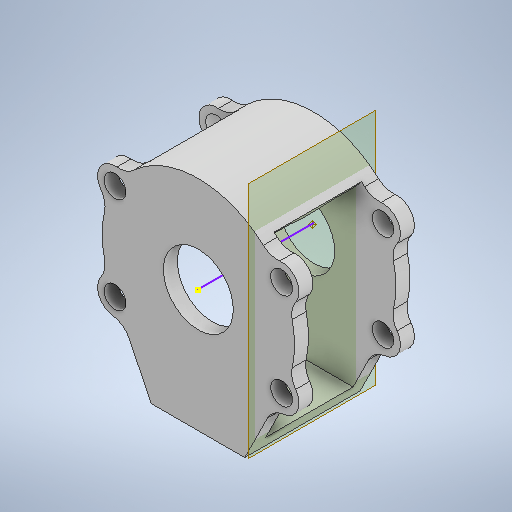
# Autodesk Inventor part: pulleyblocker
Saved by Autodesk Inventor 2025.2 (Build 292293000, 293)
## iProperties
Created: 2025-01-13
Part Number: pulleyblocker
Material: Generic
Document SubType Name: Modeling
Designer: email
Density: 1 g/cm^3
Appearance: Default
Author: email
Autodesk Inventor part; units mm, degrees
ref_plane "YZ Plane" through (0, 0, 0) normal (1, 0, 0) x (0, 1, 0)
ref_plane "XZ Plane" through (0, 0, 0) normal (0, 1, 0) x (-1, 0, 0)
ref_plane "XY Plane" through (0, 0, 0) normal (0, 0, 1) x (1, 0, 0)
sketch "Sketch1" plane through (0, 0, 0) normal (0, 0, 1) x (1, 0, 0)
  line L0 (-13.5571, -30) -> (11.7429, -30) construction
  line L1 (11.7429, -30) -> (11.7429, -13.7014) construction
  line L2 (11.7429, -13.7014) -> (-13.5571, -13.7014) construction
  line L3 (-13.5571, -13.7014) -> (-13.5571, -30) construction
  circle A0 centre (0, 0) radius 10
  circle A1 centre (0, 0) radius 23.5 construction
  line L4 (11.7429, -30) -> (21.2173, -10.1032) construction
  line L5 (-13.5571, -30) -> (-21.9053, -8.5093) construction
  circle A2 centre (0, 0) radius 27.5
  line L6 (-13.4496, -35) -> (13.2752, -35)
  line L7 (-13.4496, -35) -> (-24.6844, -12.1216)
  line L8 (13.2752, -35) -> (24.6094, -12.273)
  circle A3 centre (23.8157, 13.75) radius 5
  line L9 (-0.006, -0.0035) -> (23.8157, 13.75) construction
  line L10 (-0.006, -0.0035) -> (30.724, -0.0035) construction
  line L11 (-0.006, -0.0035) -> (23.8127, -13.7552) construction
  circle A4 centre (23.8127, -13.7552) radius 5
  circle A5 centre (23.8157, 13.75) radius 3.075
  circle A6 centre (23.8127, -13.7552) radius 3.075
  line L12 (-0.006, -0.0035) -> (-0.006, 21.9972)
  circle A7 centre (-23.8278, 13.75) radius 5
  circle A8 centre (-23.8248, -13.7552) radius 5
  circle A9 centre (-23.8278, 13.75) radius 3.075
  circle A10 centre (-23.8248, -13.7552) radius 3.075
  point P0 (20.9324, 17.8349)
  point P1 (-20.9369, 17.8296)
  point P2 (-25.9134, 9.2058)
  point P3 (-25.9114, -9.2114)
  point P4 (-21.6672, -18.2658)
  point P5 (21.6274, -18.2524)
  point P6 (25.9097, -9.2162)
  point P7 (25.9117, 9.2105)
  dimension "d0" = 25.3
  dimension "d1" = 20
  dimension "d2" = 30
  dimension "d3" = 47
  dimension "d4" = 55
  dimension "d5" = 5
  dimension "d45" = 30
  dimension "d46" = 10
  dimension "d47" = 30
  dimension "d48" = 10
  dimension "d49" = 6.15
  dimension "d50" = 6.15
  dimension "d64" = 6.15
  constraints: 26 end point, 11 centre point, 8 coincident, 6 point on circle, 4 symmetric about line, 4 tangent, 3 horizontal, 2 parallel, 1 perpendicular, 1 point on line, 1 vertical, 4 other
  measures "d0" distance between parallel lines of L1 L3
  measures "d1" diameter of A0
  measures "d2" distance from line of L0 A0.centre
  measures "d3" diameter of A1
  measures "d4" diameter of A2
  measures "d5" distance between parallel lines of L6 L0
  measures "d45" angle of L10 L9
  measures "d46" diameter of A3
  measures "d47" angle of L10 L11
  measures "d48" diameter of A4
  measures "d49" diameter of A5
  measures "d50" diameter of A6
  measures "d64" diameter of A9
extrude "Extrusion1" add sketch "Sketch1" along normal blind 4 contours A2 A4 A8 A7 A3 | A3 A2 A5 | A2 A5 A3 | A4 L8 A6 A2 | A2 A6 A4 | A4 L8 L6 L7 A8 A2 | A2 A6 L8 A4 | A7 A2 A9 | A2 A9 A7 | A8 L7 A10 A2 | A2 A10 A8 | A8 A2 A10 L7
sketch "Sketch2" plane through (0, 0, 4) normal (0, 0, 1) x (1, 0, 0)
  line L0 (-21.6672, -18.2658) -> (-13.4496, -35) projected
  line L1 (-13.4496, -35) -> (-15.4139, -31)
  line L2 (15.2701, -31) -> (-15.4139, -31)
  line L3 (13.2752, -35) -> (21.6274, -18.2524) projected
  line L4 (15.2701, -31) -> (13.2752, -35)
  line L5 (-13.4496, -35) -> (13.2752, -35) projected
  line L6 (-13.4496, -35) -> (13.2752, -35)
  point P0 (0, 0)
  point P1 (-24.6844, -12.1216)
  point P2 (24.6094, -12.273)
  dimension "d8" = 4
  constraints: 8 end point, 2 collinear, 2 point on line, 1 horizontal
  measures "d8" distance between parallel lines of L5 L2
extrude "Extrusion2" add sketch "Sketch2" along normal blind 25
sketch "Sketch3" plane through (0, 0, 29) normal (0, 0, 1) x (1, 0, 0)
  line L0 (-13.5571, -30) -> (11.7429, -30) construction
  line L1 (11.7429, -30) -> (11.7429, -13.7014) construction
  line L2 (11.7429, -13.7014) -> (-13.5571, -13.7014) construction
  line L3 (-13.5571, -13.7014) -> (-13.5571, -30) construction
  circle A0 centre (0, 0) radius 10
  circle A1 centre (0, 0) radius 23.5 construction
  line L4 (11.7429, -30) -> (21.2173, -10.1032) construction
  line L5 (-13.5571, -30) -> (-21.9053, -8.5093) construction
  circle A2 centre (0, 0) radius 27.5
  line L6 (-13.4496, -35) -> (13.2752, -35)
  line L7 (-13.4496, -35) -> (-24.6844, -12.1216)
  line L8 (13.2752, -35) -> (24.6094, -12.273)
  circle A3 centre (23.8157, 13.75) radius 5
  line L9 (-0.006, -0.0035) -> (23.8157, 13.75) construction
  line L10 (-0.006, -0.0035) -> (30.724, -0.0035) construction
  line L11 (-0.006, -0.0035) -> (23.8127, -13.7552) construction
  circle A4 centre (23.8127, -13.7552) radius 5
  circle A5 centre (23.8157, 13.75) radius 3.125
  circle A6 centre (23.8127, -13.7552) radius 3.125
  line L12 (-0.006, -0.0035) -> (-0.006, 21.9972)
  circle A7 centre (-23.8278, 13.75) radius 5
  circle A8 centre (-23.8278, 13.75) radius 3.125
  circle A9 centre (-23.8248, -13.7552) radius 5
  circle A10 centre (-23.8248, -13.7552) radius 3.125
  circle A11 centre (0, 0) radius 10 projected
  point P0 (-42.8581, 50.0798)
  point P1 (-84.7274, 50.0745)
  point P2 (-89.7039, 41.4507)
  point P3 (-89.7018, 23.0335)
  point P4 (-85.4577, 13.9792)
  point P5 (-42.163, 13.9925)
  point P6 (-37.8808, 23.0287)
  point P7 (-37.8788, 41.4554)
  point P8 (20.9324, 17.8349)
  point P9 (-20.9369, 17.8296)
  point P10 (-25.9134, 9.2058)
  point P11 (-25.9114, -9.2114)
  point P12 (-21.6672, -18.2658)
  point P13 (21.6274, -18.2524)
  point P14 (20.9285, -17.8395)
  point P15 (22.0984, -16.368)
  point P16 (25.2195, -10.9648)
  point P17 (25.9117, 9.2105)
  point P18 (25.9097, -9.2162)
  dimension "d51" = 25.3
  dimension "d52" = 20
  dimension "d53" = 30
  dimension "d54" = 47
  dimension "d55" = 55
  dimension "d56" = 5
  dimension "d57" = 30
  dimension "d58" = 10
  dimension "d59" = 30
  dimension "d60" = 10
  dimension "d61" = 6.25
  dimension "d62" = 6.25
  constraints: 26 end point, 11 centre point, 8 coincident, 6 point on circle, 4 symmetric about line, 4 tangent, 3 horizontal, 2 parallel, 1 concentric, 1 perpendicular, 1 point on line, 1 vertical, 4 other
  measures "d51" distance between parallel lines of L1 L3
  measures "d52" diameter of A0
  measures "d53" distance from line of L0 A0.centre
  measures "d54" diameter of A1
  measures "d55" diameter of A2
  measures "d56" distance between parallel lines of L6 L0
  measures "d57" angle of L10 L9
  measures "d58" diameter of A3
  measures "d59" angle of L10 L11
  measures "d60" diameter of A4
  measures "d61" diameter of A5
  measures "d62" diameter of A6
extrude "Extrusion3" add sketch "Sketch3" along normal blind 4 contours A2 A4 A9 A7 A3 | A3 A2 A5 | A2 A5 A3 | A4 L8 A6 A2 | A2 A6 A4 | A4 L8 L6 L7 A9 A2 | A2 A6 L8 A4 | A7 A2 A8 | A2 A8 A7 | A9 L7 A10 A2 | A2 A10 A9 | A9 A2 A10 L7
sketch "Sketch4" plane through (0, 0, 0) normal (1, 0, 0) x (0, 1, 0)
  line L0 (-31, 4) -> (-31, 29) projected
  line L1 (16.3793, 67.7391) -> (20.3793, 67.7391) construction
  line L2 (20.3793, 44.4757) -> (20.3793, 67.7391) construction
  line L3 (20.3793, 44.4757) -> (16.3793, 44.4757) construction
  line L4 (0, 24) -> (0, 4)
  line L5 (16.3793, 44.4757) -> (16.3793, 48.4757) construction
  line L6 (16.3793, 67.7391) -> (16.3793, 63.7391) construction
  arc A0 (16.3793, 63.7391) -> (16.3793, 48.4757) centre (22.0199, 56.1074) ccw construction
  line L7 (27.5, 4) -> (17.8296, 4) projected
  line L8 (27.5, 29) -> (27.5, 33)
  line L9 (27.5, 29) -> (-12.273, 29)
  line L10 (27.5, 29) -> (25, 29)
  line L11 (25, 29) -> (25, 22.5)
  arc A1 (25, 22.5) -> (25, 10.5) centre (31.0208, 16.5) ccw
  line L12 (25, 10.5) -> (25, 4)
  line L13 (27.5, 4) -> (25, 4)
  line L14 (25, 29) -> (27.5, 29)
  line L15 (27.5, 4) -> (27.5, 29)
  line L16 (27.5, 4) -> (17.8296, 4) projected
  line L17 (27.5, 4) -> (25, 4)
  point P0 (0, 0)
  point P1 (-12.1216, 29)
  point P2 (-12.1216, 4)
  point P3 (-12.273, 29)
  point P4 (25, 7.25)
  point P5 (17.8349, 4)
  point P6 (9.2058, 4)
  point P7 (-9.2114, 4)
  dimension "d22" = 4
  dimension "d23" = 4
  dimension "d24" = 4
  dimension "d26" = 6.5
  dimension "d28" = 6.5
  dimension "d65" = 2.5
  dimension "d66" = 2.5
  constraints: 28 end point, 4 collinear, 4 point on circle, 3 perpendicular, 3 vertical, 2 centre point, 2 point on line, 1 coincident, 1 horizontal, 1 midpoint, 4 other
  measures "d22" distance of L3.end L5.end
  measures "d23" distance of L1.start L6.end
  measures "d24" distance between parallel lines of L2 L5
  measures "d26" distance of L10.end L11.end
  measures "d28" distance of L12.start L12.end
  measures "d65" distance between parallel lines of L15 L11
  measures "d66" distance between parallel lines of L15 L12
revolve "Revolution1" add sketch "Sketch4" angle 80 mid plane about axis through (0, 0, 24) along (0, 0, -1)
sketch "Sketch5" plane through (0, 0, 0) normal (0, 1, 0) x (-1, 0, 0)
  line L0 (0, 0) -> (0.0872, 33)
  constraints: 2 end point
sketch "Sketch7" plane through (0, 0, 0) normal (1, 0, 0) x (0, 1, 0)
  line L0 (29.2747, 11.9493) -> (29.2747, 21.0264) construction
  ellipse E0 centre (23.7633, 16.5) end of major axis (23.7633, 8) minor radius 6.5114 (19.1511, 22.5) -> (19.1511, 10.5) ccw projected
  line L1 (29.2747, 16.4878) -> (30.2747, 16.4878)
  arc A0 (29.2747, 11.9493) -> (29.2747, 21.0264) centre (45.8325, 16.4878) ccw
  arc A1 (30.2415, 15.6424) -> (30.2747, 16.4878) centre (23.4449, 16.3328) ccw
  line L2 (29.2747, 21.0264) -> (27.6139, 21.0264)
  line L3 (27.6139, 21.0264) -> (27.6139, 13.9093)
  line L4 (27.6139, 13.9093) -> (29.2747, 13.9093)
  line L5 (29.2747, 13.9093) -> (29.2747, 21.0264)
  point P0 (0, 0)
  point P1 (13.8599, 14.7128)
  point P2 (13.8237, 14.0101)
  point P3 (14.8237, 10.4516)
  dimension "d29" = 1
  constraints: 12 end point, 4 point on circle, 2 centre point, 2 horizontal, 2 parallel, 1 midpoint, 1 perpendicular, 1 vertical, 4 other
  measures "d29" distance of L1.end L1.start
extrude "Extrusion4" [suppressed]
sketch "Sketch9" plane through (-13.4496, -35, 0) normal (0, -1, 0) x (1, 0, 0)
  circle A0 centre (13.3624, 16.5) radius 5
  line L0 (0, 33) -> (26.7249, 33)
  line L1 (0, 0) -> (0, 29) projected
  line L2 (26.7249, 0) -> (26.7249, 29) projected
  line L3 (0, 0) -> (26.7249, 0) projected
  point P0 (13.4496, 0)
  dimension "d34" = 16.5
  dimension "d35" = 13.3624
  dimension "d36" = 26.7249
  dimension "d37" = 10
  dimension "d44" = 33
  constraints: 2 end point, 1 centre point
  measures "d34" distance from line of L0 A0.centre
  measures "d35" distance from line of L1 A0.centre
  measures "d36" distance between parallel lines of L1 L2
  measures "d37" diameter of A0
  measures "d44" distance between parallel lines of L3 L0
extrude "Extrusion5" cut sketch "Sketch9" against normal up to surface (4 mm away)
ref_plane "Work Plane1" through (16.0697, 19.1511, 29) normal (-1, 0, 0) x (0, 0, -1)
sketch "Sketch11" plane through (0, 0, 33) normal (0, 0, 1) x (1, 0, 0)
  point P0 (0, 0)
fillet "Fillet3" radius 6 14 edges at (20.9324, 17.8349, 31) (20.9324, 17.8349, 2) (25.9117, 9.2105, 31) (25.9117, 9.2105, 2) (25.9097, -9.2162, 2) (21.6274, -18.2524, 2) (-25.9134, 9.2058, 31) (-25.9134, 9.2058, 2) (-20.9369, 17.8296, 2) (-20.9369, 17.8296, 31) (-25.9114, -9.2114, 31) (-21.6672, -18.2658, 31) (25.9097, -9.2162, 31) (21.6274, -18.2524, 31)
equation "\"d35\" = 0.5 * d36"
body "Solid1"
